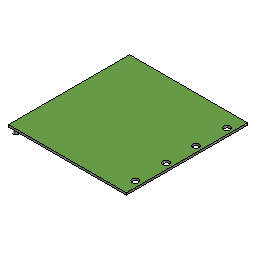
Placa teren Dreapta (Autodesk Fusion 360 design; units mm, degrees)
part number: 2026-06-02-22-20-53-798
Autodesk Fusion 360 part; units mm, degrees
sketch "Sketch1" plane through (0, 0, 0) normal (0, 0, 1) x (1, 0, 0)
  line L0 (46.8447, 156.9249) -> (-67.5, 156.9249)
  line L1 (-67.5, 156.9249) -> (-67.5, 42.5803)
  line L2 (43.8447, 42.5803) -> (43.8447, 156.9249)
  line L3 (-67.5, 42.5803) -> (46.8447, 42.5803)
  circle A0 centre (38.3447, 142.9249) radius 3
  circle A1 centre (38.3447, 113.7526) radius 3
  circle A2 centre (38.3447, 85.7526) radius 3
  circle A3 centre (38.3447, 56.5803) radius 3
  circle A4 centre (-10.3277, 59.7526) radius 2
  circle A5 centre (-64, 46.0803) radius 2
  circle A6 centre (-64, 82.2526) radius 2
  circle A7 centre (-10.3277, 99.7526) radius 2
  circle A8 centre (-10.3277, 139.7526) radius 2
  circle A9 centre (-64, 153.4249) radius 2
  circle A10 centre (-64, 117.2526) radius 2
  dimension "d687" = 6
  dimension "d688" = 4
  dimension "d689" = 10.3277
  dimension "d690" = 54.1723
  dimension "d691" = 53.6723
  dimension "d692" = 48.6723
  dimension "d693" = 114.3447
  dimension "d694" = 57.1723
  dimension "d695" = 17.1723
  dimension "d696" = 97.1723
  dimension "d697" = 57.1723
  dimension "d698" = 59.7526
  dimension "d699" = 93.6723
  dimension "d700" = 83.1723
  dimension "d701" = 80
  dimension "d702" = 57.5
  dimension "d703" = 54
  dimension "d704" = 26
  dimension "d705" = 22.5
  dimension "d706" = 13.6723
  dimension "d707" = 3.1723
  constraint coincident L2.start L3
  constraint coincident L0 L2.end
  constraint vertical L1
  constraint vertical L2
  constraint horizontal L3
  constraint horizontal L0
  constraint vertical A5.centre A6.centre
  constraint vertical A5.centre A10.centre
  constraint vertical A5.centre A9.centre
  constraint vertical A4.centre A7.centre
  constraint vertical A4.centre A8.centre
  constraint vertical A2.centre A3.centre
  constraint vertical A1.centre A3.centre
  constraint vertical A0.centre A3.centre
  constraint equal A4 A5
  constraint equal A4 A6
  constraint equal A4 A7
  constraint equal A4 A8
  constraint equal A4 A9
  constraint equal A4 A10
  constraint equal A0 A1
  constraint equal A0 A2
  constraint equal A0 A3
  constraint equal L0 L2
  measures "d687" diameter of A1
  measures "d688" diameter of A4
  measures "d689" horizontal distance of origin A4.centre
  measures "d690" distance of L2 A4.centre
  measures "d691" horizontal distance of A4.centre A5.centre
  measures "d692" horizontal distance of A3.centre A4.centre
  measures "d693" horizontal distance of L1.end L3.end
  measures "d694" distance of L1 A8.centre
  measures "d695" distance of L3 A4.centre
  measures "d696" distance of L0 A4.centre
  measures "d697" vertical distance of L3.end A7.centre
  measures "d698" vertical distance of origin A4.centre
  measures "d699" vertical distance of A4.centre A9.centre
  measures "d700" vertical distance of A0.centre A4.centre
  measures "d701" vertical distance of A4.centre A8.centre
  measures "d702" vertical distance of A4.centre A10.centre
  measures "d703" vertical distance of A1.centre A4.centre
  measures "d704" vertical distance of A2.centre A4.centre
  measures "d705" vertical distance of A4.centre A6.centre
  measures "d706" vertical distance of A4.centre A5.centre
  measures "d707" vertical distance of A3.centre A4.centre
extrude "Extrude1" add sketch "Sketch1" along normal blind 2 contours L0 L1 L2 L3 | A4 | A5 | A6 | A7 | A8 | A9 | A10
extrude "Extrude2" add sketch "Sketch1" against normal blind 5 contours A4 | A5 | A6 | A7 | A8 | A9 | A10
